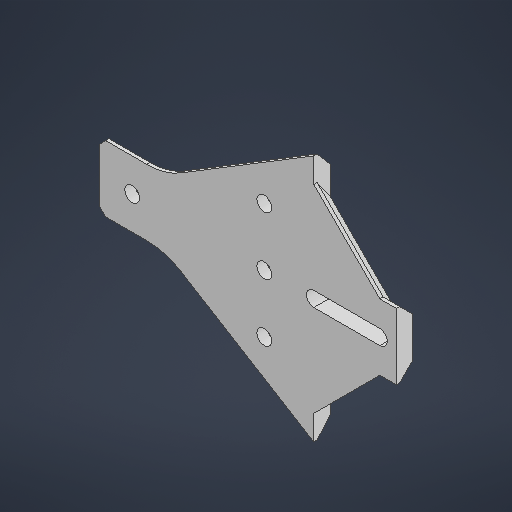
# Autodesk Inventor part: Y Axis Bearing Holder
Saved by Autodesk Inventor 2025.1 (Build 291241000, 241)
## iProperties
Created: 2025-02-22
Part Number: Y Axis Bearing Holder
Material: Generic
Document SubType Name: Modeling
Designer: jerem
Density: 1 g/cm^3
Appearance: Default
Author: jerem
## iProperties of the stored document Y Axis Bearing Holder_3DPrint.ipt
Created: 2025-02-22
Part Number: Y Axis Bearing Holder_3DPrint
Material: Generic
Document SubType Name: Modeling
Designer: jerem
Density: 1 g/cm^3
Appearance: Default
Author: jerem
Autodesk Inventor part; units mm, degrees
ref_plane "YZ Plane" through (0, 0, 0) normal (1, 0, 0) x (0, 1, 0)
ref_plane "XZ Plane" through (0, 0, 0) normal (0, 1, 0) x (-1, 0, 0)
ref_plane "XY Plane" through (0, 0, 0) normal (0, 0, 1) x (1, 0, 0)
sketch "Sketch1" plane through (0, 0, 0) normal (0, 0, 1) x (1, 0, 0)
  line L0 (0, 0) -> (-50, 0) construction
  line L1 (-50, 0) -> (-50, 10)
  line L2 (-50, 0) -> (-50, -10)
  line L3 (-50, -10) -> (-30, -10)
  line L4 (-30, -10) -> (15, -37.5)
  line L5 (-50, 10) -> (-30, 10)
  line L6 (-30, 10) -> (15, 37.5)
  line L7 (15, 37.5) -> (15, -37.5)
  line L8 (0, 0) -> (15, 0) construction
  line L9 (0, 17.5) -> (0, -17.5) construction
  line L10 (-30, 10) -> (40, 10)
  line L11 (-30, -10) -> (40, -10)
  line L12 (40, 10) -> (40, -10)
  circle A0 centre (35, 0) radius 2.25
  circle A1 centre (15, 0) radius 2.25
  line L13 (35, 2.25) -> (15, 2.25)
  line L14 (15, -2.25) -> (35, -2.25)
  point P0 (-40, 0)
  point P1 (40, 0)
  point P2 (15, -10)
  point P3 (15, 10)
  dimension "d0" = 20
  dimension "d1" = 65
  dimension "d2" = 50
  dimension "d4" = 20
  dimension "d5" = 75
  dimension "d6" = 35
  dimension "d9" = 40
  dimension "d21" = 25
  dimension "d22" = 5
  dimension "d23" = 4.5
  constraints: 30 end point, 4 coincident, 4 horizontal, 4 point on circle, 4 vertical, 3 equal length, 3 midpoint, 3 point on line, 3 tangent, 2 centre point, 2 perpendicular, 1 equal radius
  measures "d0" distance between parallel lines of L3 L5
  measures "d1" distance of L8.end L0.end
  measures "d2" distance between parallel lines of L1 L9
  measures "d4" distance of L1.end L5.end
  measures "d5" distance of L6.end L4.end
  measures "d6" distance of L9.end L9.start
  measures "d9" distance of L0.start point (-40, 0)
  measures "d21" distance between parallel lines of L7 L12
  measures "d22" distance of point (40, 0) A0.centre
  measures "d23" diameter of A0
extrude "Extrusion1" add sketch "Sketch1" along normal blind 5 contours L1 L5 L10 L7 A1 L11 L3 L2 | L6 L7 L10 | L11 L7 L4 | L10 L12 L11 L7 L14 A0 L13
hole "Hole1" at (0, 17.5, 0) at (0, -17.5, 0) at (-40, 0, 0) at (0, 0, 0) direction (0, 0, 1) diameter 4.5 end through all counterbore diameter 8 counterbore depth 2
fillet "Fillet1" radius 20 2 edges at (-30, 10, 2.5) (-30, -10, 2.5)
chamfer "Chamfer1" distance 2 angle 45 2 edges at (-50, 10, 2.5) (-50, -10, 2.5)
chamfer "Chamfer2" distance 20 angle 45 2 edges at (15, 10, 2.5) (15, -10, 2.5)
chamfer "Chamfer3" distance 4 angle 45 10 edges at (-5.0992, 25.2172, 0) (-30.2103, 10.7476, 0) (-41.8137, 10, 0) (-41.8137, -10, 0) (-30.2103, -10.7476, 0) (-5.0992, -25.2172, 0) (37.5, 10, 0) (25, 20, 0) (37.5, -10, 0) (25, -20, 0)
body "Solid1"
